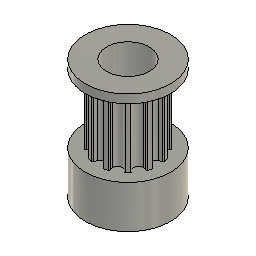
c7a76a11-5d82-49f7-98bc-9a9dc2cbd4a3 (Autodesk Fusion 360 design; units mm, degrees)
Autodesk Fusion 360 part; units mm, degrees
sketch "Sketch1" plane through (0, 0, 0) normal (0, 0, 1) x (1, 0, 0)
  arc A0 (6.2495, 2.4169) -> (6.267, 1.8336) centre (6.7302, 2.1394) ccw
  arc A1 (2.6934, 6.7634) -> (2.6052, 7.0865) centre (1.6982, 6.6655) ccw
  arc A2 (6.9322, 3.3233) -> (7.2561, 3.2381) centre (7.345, 4.2342) ccw
  arc A3 (2.4169, 1.3899) -> (1.8336, 1.3724) centre (2.1394, 0.9093) ccw
  arc A4 (3.3233, 6.9322) -> (3.8197, 6.6254) centre (3.8197, 7.1804) ccw
  arc A5 (6.2357, 6.5436) -> (6.0416, 6.5049) centre (6.1607, 6.4137) ccw
  arc A6 (4.9707, 0.3655) -> (5.0342, 0.5529) centre (4.8957, 0.4954) ccw
  arc A7 (0.5529, 5.0342) -> (0.3655, 4.9707) centre (0.4954, 4.8957) ccw
  arc A8 (3.0894, 7.3867) -> (2.6687, 7.274) centre (3.8002, 3.8925) ccw
  arc A9 (6.2495, 5.2226) -> (6.7634, 4.9461) centre (6.7302, 5.5001) ccw
  arc A10 (3.0894, 0.2527) -> (3.2381, 0.3833) centre (3.0894, 0.4027) ccw
  arc A11 (7.2561, 4.4013) -> (6.9322, 4.3161) centre (7.345, 3.4053) ccw
  arc A12 (4.4013, 0.3833) -> (4.3161, 0.7072) centre (3.4053, 0.2945) ccw
  arc A13 (7.3867, 4.5501) -> (7.274, 4.9707) centre (3.8925, 3.8392) ccw
  arc A14 (4.3161, 6.9322) -> (4.4013, 7.2561) centre (3.4053, 7.345) ccw
  arc A15 (1.8336, 1.3724) -> (1.5978, 1.1345) centre (2.416, 0.5595) ccw
  arc A16 (1.3724, 5.8059) -> (1.1345, 6.0416) centre (0.5595, 5.2234) ccw
  arc A17 (3.8197, 1.014) -> (3.3233, 0.7072) centre (3.8197, 0.459) ccw
  arc A18 (1.0958, 1.4037) -> (1.4037, 1.0958) centre (3.7664, 3.7664) ccw
  arc A19 (0.876, 2.6934) -> (0.5529, 2.6052) centre (0.974, 1.6982) ccw
  arc A20 (4.5501, 7.3867) -> (4.4013, 7.2561) centre (4.5501, 7.2367) ccw
  arc A21 (5.0342, 7.0865) -> (4.9707, 7.274) centre (4.8957, 7.1441) ccw
  arc A22 (3.2381, 7.2561) -> (3.0894, 7.3867) centre (3.0894, 7.2367) ccw
  arc A23 (1.1345, 1.5978) -> (1.3724, 1.8336) centre (0.5595, 2.416) ccw
  arc A24 (6.2357, 1.0958) -> (6.5436, 1.4037) centre (3.873, 3.7664) ccw
  arc A25 (2.6052, 0.5529) -> (2.6687, 0.3655) centre (2.7437, 0.4954) ccw
  arc A26 (1.0958, 6.2357) -> (1.1345, 6.0416) centre (1.2257, 6.1607) ccw
  arc A27 (3.3233, 0.7072) -> (3.2381, 0.3833) centre (4.2342, 0.2945) ccw
  arc A28 (1.4037, 6.5436) -> (1.0958, 6.2357) centre (3.7664, 3.873) ccw
  arc A29 (6.7634, 4.9461) -> (7.0865, 5.0342) centre (6.6655, 5.9413) ccw
  arc A30 (4.9461, 6.7634) -> (5.2226, 6.2495) centre (5.5001, 6.7302) ccw
  arc A31 (1.014, 3.8197) -> (0.7072, 4.3161) centre (0.459, 3.8197) ccw
  arc A32 (6.9322, 4.3161) -> (6.6254, 3.8197) centre (7.1804, 3.8197) ccw
  arc A33 (3.8197, 6.6254) -> (4.3161, 6.9322) centre (3.8197, 7.1804) ccw
  arc A34 (6.6254, 3.8197) -> (6.9322, 3.3233) centre (7.1804, 3.8197) ccw
  arc A35 (1.3899, 5.2226) -> (1.3724, 5.8059) centre (0.9093, 5.5001) ccw
  arc A36 (2.6934, 0.876) -> (2.4169, 1.3899) centre (2.1394, 0.9093) ccw
  arc A37 (0.5529, 5.0342) -> (0.876, 4.9461) centre (0.974, 5.9413) ccw
  arc A38 (1.3724, 1.8336) -> (1.3899, 2.4169) centre (0.9093, 2.1394) ccw
  arc A39 (0.3655, 2.6687) -> (0.5529, 2.6052) centre (0.4954, 2.7437) ccw
  arc A40 (1.5978, 6.5049) -> (1.8336, 6.267) centre (2.416, 7.0799) ccw
  arc A41 (6.5436, 1.4037) -> (6.5049, 1.5978) centre (6.4137, 1.4787) ccw
  arc A42 (0.3655, 4.9707) -> (0.2527, 4.5501) centre (3.7469, 3.8392) ccw
  arc A43 (7.274, 2.6687) -> (7.3867, 3.0894) centre (3.8925, 3.8002) ccw
  arc A44 (7.3867, 3.0894) -> (7.2561, 3.2381) centre (7.2367, 3.0894) ccw
  arc A45 (0.3833, 3.2381) -> (0.7072, 3.3233) centre (0.2945, 4.2342) ccw
  arc A46 (7.0865, 2.6052) -> (7.274, 2.6687) centre (7.1441, 2.7437) ccw
  arc A47 (0.7072, 4.3161) -> (0.3833, 4.4013) centre (0.2945, 3.4053) ccw
  arc A48 (7.2561, 4.4013) -> (7.3867, 4.5501) centre (7.2367, 4.5501) ccw
  arc A49 (5.0342, 7.0865) -> (4.9461, 6.7634) centre (5.9413, 6.6655) ccw
  arc A50 (7.0865, 2.6052) -> (6.7634, 2.6934) centre (6.6655, 1.6982) ccw
  arc A51 (4.5501, 0.2527) -> (4.9707, 0.3655) centre (3.8392, 3.7469) ccw
  arc A52 (6.7634, 2.6934) -> (6.2495, 2.4169) centre (6.7302, 2.1394) ccw
  arc A53 (5.2226, 6.2495) -> (5.8059, 6.267) centre (5.5001, 6.7302) ccw
  arc A54 (1.8336, 6.267) -> (2.4169, 6.2495) centre (2.1394, 6.7302) ccw
  arc A55 (4.9461, 0.876) -> (5.0342, 0.5529) centre (5.9413, 0.974) ccw
  circle A56 centre (3.8197, 3.8197) radius 2.5
  arc A57 (0.3833, 3.2381) -> (0.2527, 3.0894) centre (0.4027, 3.0894) ccw
  arc A58 (0.2527, 3.0894) -> (0.3655, 2.6687) centre (3.7469, 3.8002) ccw
  arc A59 (4.9707, 7.274) -> (4.5501, 7.3867) centre (3.8392, 3.8925) ccw
  arc A60 (6.0416, 1.1345) -> (5.8059, 1.3724) centre (5.2234, 0.5595) ccw
  arc A61 (4.4013, 0.3833) -> (4.5501, 0.2527) centre (4.5501, 0.4027) ccw
  arc A62 (1.1345, 1.5978) -> (1.0958, 1.4037) centre (1.2257, 1.4787) ccw
  arc A63 (3.2381, 7.2561) -> (3.3233, 6.9322) centre (4.2342, 7.345) ccw
  arc A64 (7.274, 4.9707) -> (7.0865, 5.0342) centre (7.1441, 4.8957) ccw
  arc A65 (6.267, 1.8336) -> (6.5049, 1.5978) centre (7.0799, 2.416) ccw
  arc A66 (4.3161, 0.7072) -> (3.8197, 1.014) centre (3.8197, 0.459) ccw
  arc A67 (0.2527, 4.5501) -> (0.3833, 4.4013) centre (0.4027, 4.5501) ccw
  arc A68 (1.5978, 6.5049) -> (1.4037, 6.5436) centre (1.4787, 6.4137) ccw
  arc A69 (6.267, 5.8059) -> (6.2495, 5.2226) centre (6.7302, 5.5001) ccw
  arc A70 (5.8059, 6.267) -> (6.0416, 6.5049) centre (5.2234, 7.0799) ccw
  arc A71 (0.876, 4.9461) -> (1.3899, 5.2226) centre (0.9093, 5.5001) ccw
  arc A72 (6.5436, 6.2357) -> (6.2357, 6.5436) centre (3.873, 3.873) ccw
  arc A73 (6.5049, 6.0416) -> (6.267, 5.8059) centre (7.0799, 5.2234) ccw
  arc A74 (1.3899, 2.4169) -> (0.876, 2.6934) centre (0.9093, 2.1394) ccw
  arc A75 (6.0416, 1.1345) -> (6.2357, 1.0958) centre (6.1607, 1.2257) ccw
  arc A76 (2.6687, 7.274) -> (2.6052, 7.0865) centre (2.7437, 7.1441) ccw
  arc A77 (6.5049, 6.0416) -> (6.5436, 6.2357) centre (6.4137, 6.1607) ccw
  arc A78 (0.7072, 3.3233) -> (1.014, 3.8197) centre (0.459, 3.8197) ccw
  arc A79 (2.6052, 0.5529) -> (2.6934, 0.876) centre (1.6982, 0.974) ccw
  arc A80 (5.8059, 1.3724) -> (5.2226, 1.3899) centre (5.5001, 0.9093) ccw
  arc A81 (5.2226, 1.3899) -> (4.9461, 0.876) centre (5.5001, 0.9093) ccw
  arc A82 (1.4037, 1.0958) -> (1.5978, 1.1345) centre (1.4787, 1.2257) ccw
  arc A83 (2.4169, 6.2495) -> (2.6934, 6.7634) centre (2.1394, 6.7302) ccw
  arc A84 (2.6687, 0.3655) -> (3.0894, 0.2527) centre (3.8002, 3.7469) ccw
extrude "Extrude1" add sketch "Sketch1" along normal blind 8
sketch "Sketch2" plane through (0, 0, 8) normal (0, 0, 1) x (-1, 0, 0)
  circle A0 centre (-3.8197, -3.8197) radius 2.5
  arc A1 (-2.6052, -0.5529) -> (-2.6687, -0.3655) centre (-2.7437, -0.4954) ccw
  arc A2 (-2.6687, -0.3655) -> (-3.0894, -0.2527) centre (-3.8002, -3.7469) ccw
  arc A3 (-3.0894, -0.2527) -> (-3.2381, -0.3833) centre (-3.0894, -0.4027) ccw
  arc A4 (-3.3233, -0.7072) -> (-3.2381, -0.3833) centre (-4.2342, -0.2945) ccw
  arc A5 (-4.3161, -0.7072) -> (-3.3233, -0.7072) centre (-3.8197, -0.459) ccw
  arc A6 (-4.4013, -0.3833) -> (-4.3161, -0.7072) centre (-3.4053, -0.2945) ccw
  arc A7 (-4.4013, -0.3833) -> (-4.5501, -0.2527) centre (-4.5501, -0.4027) ccw
  arc A8 (-4.5501, -0.2527) -> (-4.9707, -0.3655) centre (-3.8392, -3.7469) ccw
  arc A9 (-4.9707, -0.3655) -> (-5.0342, -0.5529) centre (-4.8957, -0.4954) ccw
  arc A10 (-4.9461, -0.876) -> (-5.0342, -0.5529) centre (-5.9413, -0.974) ccw
  arc A11 (-5.8059, -1.3724) -> (-4.9461, -0.876) centre (-5.5001, -0.9093) ccw
  arc A12 (-6.0416, -1.1345) -> (-5.8059, -1.3724) centre (-5.2234, -0.5595) ccw
  arc A13 (-6.0416, -1.1345) -> (-6.2357, -1.0958) centre (-6.1607, -1.2257) ccw
  arc A14 (-6.2357, -1.0958) -> (-6.5436, -1.4037) centre (-3.873, -3.7664) ccw
  arc A15 (-6.5436, -1.4037) -> (-6.5049, -1.5978) centre (-6.4137, -1.4787) ccw
  arc A16 (-6.267, -1.8336) -> (-6.5049, -1.5978) centre (-7.0799, -2.416) ccw
  arc A17 (-6.7634, -2.6934) -> (-6.267, -1.8336) centre (-6.7302, -2.1394) ccw
  arc A18 (-7.0865, -2.6052) -> (-6.7634, -2.6934) centre (-6.6655, -1.6982) ccw
  arc A19 (-7.0865, -2.6052) -> (-7.274, -2.6687) centre (-7.1441, -2.7437) ccw
  arc A20 (-7.274, -2.6687) -> (-7.3867, -3.0894) centre (-3.8925, -3.8002) ccw
  arc A21 (-7.3867, -3.0894) -> (-7.2561, -3.2381) centre (-7.2367, -3.0894) ccw
  arc A22 (-6.9322, -3.3233) -> (-7.2561, -3.2381) centre (-7.345, -4.2342) ccw
  arc A23 (-6.9322, -4.3161) -> (-6.9322, -3.3233) centre (-7.1804, -3.8197) ccw
  arc A24 (-7.2561, -4.4013) -> (-6.9322, -4.3161) centre (-7.345, -3.4053) ccw
  arc A25 (-7.2561, -4.4013) -> (-7.3867, -4.5501) centre (-7.2367, -4.5501) ccw
  arc A26 (-7.3867, -4.5501) -> (-7.274, -4.9707) centre (-3.8925, -3.8392) ccw
  arc A27 (-7.274, -4.9707) -> (-7.0865, -5.0342) centre (-7.1441, -4.8957) ccw
  arc A28 (-6.7634, -4.9461) -> (-7.0865, -5.0342) centre (-6.6655, -5.9413) ccw
  arc A29 (-6.267, -5.8059) -> (-6.7634, -4.9461) centre (-6.7302, -5.5001) ccw
  arc A30 (-6.5049, -6.0416) -> (-6.267, -5.8059) centre (-7.0799, -5.2234) ccw
  arc A31 (-6.5049, -6.0416) -> (-6.5436, -6.2357) centre (-6.4137, -6.1607) ccw
  arc A32 (-6.5436, -6.2357) -> (-6.2357, -6.5436) centre (-3.873, -3.873) ccw
  arc A33 (-6.2357, -6.5436) -> (-6.0416, -6.5049) centre (-6.1607, -6.4137) ccw
  arc A34 (-5.8059, -6.267) -> (-6.0416, -6.5049) centre (-5.2234, -7.0799) ccw
  arc A35 (-4.9461, -6.7634) -> (-5.8059, -6.267) centre (-5.5001, -6.7302) ccw
  arc A36 (-5.0342, -7.0865) -> (-4.9461, -6.7634) centre (-5.9413, -6.6655) ccw
  arc A37 (-5.0342, -7.0865) -> (-4.9707, -7.274) centre (-4.8957, -7.1441) ccw
  arc A38 (-4.9707, -7.274) -> (-4.5501, -7.3867) centre (-3.8392, -3.8925) ccw
  arc A39 (-4.5501, -7.3867) -> (-4.4013, -7.2561) centre (-4.5501, -7.2367) ccw
  arc A40 (-4.3161, -6.9322) -> (-4.4013, -7.2561) centre (-3.4053, -7.345) ccw
  arc A41 (-3.3233, -6.9322) -> (-4.3161, -6.9322) centre (-3.8197, -7.1804) ccw
  arc A42 (-3.2381, -7.2561) -> (-3.3233, -6.9322) centre (-4.2342, -7.345) ccw
  arc A43 (-3.2381, -7.2561) -> (-3.0894, -7.3867) centre (-3.0894, -7.2367) ccw
  arc A44 (-3.0894, -7.3867) -> (-2.6687, -7.274) centre (-3.8002, -3.8925) ccw
  arc A45 (-2.6687, -7.274) -> (-2.6052, -7.0865) centre (-2.7437, -7.1441) ccw
  arc A46 (-2.6934, -6.7634) -> (-2.6052, -7.0865) centre (-1.6982, -6.6655) ccw
  arc A47 (-1.8336, -6.267) -> (-2.6934, -6.7634) centre (-2.1394, -6.7302) ccw
  arc A48 (-1.5978, -6.5049) -> (-1.8336, -6.267) centre (-2.416, -7.0799) ccw
  arc A49 (-1.5978, -6.5049) -> (-1.4037, -6.5436) centre (-1.4787, -6.4137) ccw
  arc A50 (-1.4037, -6.5436) -> (-1.0958, -6.2357) centre (-3.7664, -3.873) ccw
  arc A51 (-1.0958, -6.2357) -> (-1.1345, -6.0416) centre (-1.2257, -6.1607) ccw
  arc A52 (-1.3724, -5.8059) -> (-1.1345, -6.0416) centre (-0.5595, -5.2234) ccw
  arc A53 (-0.876, -4.9461) -> (-1.3724, -5.8059) centre (-0.9093, -5.5001) ccw
  arc A54 (-0.5529, -5.0342) -> (-0.876, -4.9461) centre (-0.974, -5.9413) ccw
  arc A55 (-0.5529, -5.0342) -> (-0.3655, -4.9707) centre (-0.4954, -4.8957) ccw
  arc A56 (-0.3655, -4.9707) -> (-0.2527, -4.5501) centre (-3.7469, -3.8392) ccw
  arc A57 (-0.2527, -4.5501) -> (-0.3833, -4.4013) centre (-0.4027, -4.5501) ccw
  arc A58 (-0.7072, -4.3161) -> (-0.3833, -4.4013) centre (-0.2945, -3.4053) ccw
  arc A59 (-0.7072, -3.3233) -> (-0.7072, -4.3161) centre (-0.459, -3.8197) ccw
  arc A60 (-0.3833, -3.2381) -> (-0.7072, -3.3233) centre (-0.2945, -4.2342) ccw
  arc A61 (-0.3833, -3.2381) -> (-0.2527, -3.0894) centre (-0.4027, -3.0894) ccw
  arc A62 (-0.2527, -3.0894) -> (-0.3655, -2.6687) centre (-3.7469, -3.8002) ccw
  arc A63 (-0.3655, -2.6687) -> (-0.5529, -2.6052) centre (-0.4954, -2.7437) ccw
  arc A64 (-0.876, -2.6934) -> (-0.5529, -2.6052) centre (-0.974, -1.6982) ccw
  arc A65 (-1.3724, -1.8336) -> (-0.876, -2.6934) centre (-0.9093, -2.1394) ccw
  arc A66 (-1.1345, -1.5978) -> (-1.3724, -1.8336) centre (-0.5595, -2.416) ccw
  arc A67 (-1.1345, -1.5978) -> (-1.0958, -1.4037) centre (-1.2257, -1.4787) ccw
  arc A68 (-1.0958, -1.4037) -> (-1.4037, -1.0958) centre (-3.7664, -3.7664) ccw
  arc A69 (-1.4037, -1.0958) -> (-1.5978, -1.1345) centre (-1.4787, -1.2257) ccw
  arc A70 (-1.8336, -1.3724) -> (-1.5978, -1.1345) centre (-2.416, -0.5595) ccw
  arc A71 (-2.6934, -0.876) -> (-1.8336, -1.3724) centre (-2.1394, -0.9093) ccw
  arc A72 (-2.6052, -0.5529) -> (-2.6934, -0.876) centre (-1.6982, -0.974) ccw
  circle A73 centre (-3.8197, -3.8197) radius 5
  dimension "d3" = 10
  constraint concentric A0 A73
  measures "d3" diameter of A73
extrude "Extrude2" add sketch "Sketch2" along normal blind 1 contours A1 A2 A3 A4 A5 A6 A7 A8 A9 A10 A11 A12 A13 A14 A15 A16 A17 A18 A19 A20 A21 A22 A23 A24 A25 A26 A27 A28 A29 A30 A31 A32 A33 A34 A35 A36 A37 A38 A39 A40 A41 A42 A43 A44 A45 A46 A47 A48 A49 A50 A51 A52 A53 A54 A55 A56 A57 A58 A59 A60 A61 A62 A63 A64 A65 A66 A67 A68 A69 A70 A71 A72 | A73
sketch "Sketch3" plane through (0, 0, 0) normal (0, 0, -1) x (1, 0, 0)
  circle A0 centre (3.8197, -3.8197) radius 2.5
  arc A1 (2.6687, -0.3655) -> (2.6052, -0.5529) centre (2.7437, -0.4954) ccw
  arc A2 (2.6934, -0.876) -> (2.6052, -0.5529) centre (1.6982, -0.974) ccw
  arc A3 (1.8336, -1.3724) -> (2.6934, -0.876) centre (2.1394, -0.9093) ccw
  arc A4 (1.5978, -1.1345) -> (1.8336, -1.3724) centre (2.416, -0.5595) ccw
  arc A5 (1.5978, -1.1345) -> (1.4037, -1.0958) centre (1.4787, -1.2257) ccw
  arc A6 (1.4037, -1.0958) -> (1.0958, -1.4037) centre (3.7664, -3.7664) ccw
  arc A7 (1.0958, -1.4037) -> (1.1345, -1.5978) centre (1.2257, -1.4787) ccw
  arc A8 (1.3724, -1.8336) -> (1.1345, -1.5978) centre (0.5595, -2.416) ccw
  arc A9 (0.876, -2.6934) -> (1.3724, -1.8336) centre (0.9093, -2.1394) ccw
  arc A10 (0.5529, -2.6052) -> (0.876, -2.6934) centre (0.974, -1.6982) ccw
  arc A11 (0.5529, -2.6052) -> (0.3655, -2.6687) centre (0.4954, -2.7437) ccw
  arc A12 (0.3655, -2.6687) -> (0.2527, -3.0894) centre (3.7469, -3.8002) ccw
  arc A13 (0.2527, -3.0894) -> (0.3833, -3.2381) centre (0.4027, -3.0894) ccw
  arc A14 (0.7072, -3.3233) -> (0.3833, -3.2381) centre (0.2945, -4.2342) ccw
  arc A15 (0.7072, -4.3161) -> (0.7072, -3.3233) centre (0.459, -3.8197) ccw
  arc A16 (0.3833, -4.4013) -> (0.7072, -4.3161) centre (0.2945, -3.4053) ccw
  arc A17 (0.3833, -4.4013) -> (0.2527, -4.5501) centre (0.4027, -4.5501) ccw
  arc A18 (0.2527, -4.5501) -> (0.3655, -4.9707) centre (3.7469, -3.8392) ccw
  arc A19 (0.3655, -4.9707) -> (0.5529, -5.0342) centre (0.4954, -4.8957) ccw
  arc A20 (0.876, -4.9461) -> (0.5529, -5.0342) centre (0.974, -5.9413) ccw
  arc A21 (1.3724, -5.8059) -> (0.876, -4.9461) centre (0.9093, -5.5001) ccw
  arc A22 (1.1345, -6.0416) -> (1.3724, -5.8059) centre (0.5595, -5.2234) ccw
  arc A23 (1.1345, -6.0416) -> (1.0958, -6.2357) centre (1.2257, -6.1607) ccw
  arc A24 (1.0958, -6.2357) -> (1.4037, -6.5436) centre (3.7664, -3.873) ccw
  arc A25 (1.4037, -6.5436) -> (1.5978, -6.5049) centre (1.4787, -6.4137) ccw
  arc A26 (1.8336, -6.267) -> (1.5978, -6.5049) centre (2.416, -7.0799) ccw
  arc A27 (2.6934, -6.7634) -> (1.8336, -6.267) centre (2.1394, -6.7302) ccw
  arc A28 (2.6052, -7.0865) -> (2.6934, -6.7634) centre (1.6982, -6.6655) ccw
  arc A29 (2.6052, -7.0865) -> (2.6687, -7.274) centre (2.7437, -7.1441) ccw
  arc A30 (2.6687, -7.274) -> (3.0894, -7.3867) centre (3.8002, -3.8925) ccw
  arc A31 (3.0894, -7.3867) -> (3.2381, -7.2561) centre (3.0894, -7.2367) ccw
  arc A32 (3.3233, -6.9322) -> (3.2381, -7.2561) centre (4.2342, -7.345) ccw
  arc A33 (4.3161, -6.9322) -> (3.3233, -6.9322) centre (3.8197, -7.1804) ccw
  arc A34 (4.4013, -7.2561) -> (4.3161, -6.9322) centre (3.4053, -7.345) ccw
  arc A35 (4.4013, -7.2561) -> (4.5501, -7.3867) centre (4.5501, -7.2367) ccw
  arc A36 (4.5501, -7.3867) -> (4.9707, -7.274) centre (3.8392, -3.8925) ccw
  arc A37 (4.9707, -7.274) -> (5.0342, -7.0865) centre (4.8957, -7.1441) ccw
  arc A38 (4.9461, -6.7634) -> (5.0342, -7.0865) centre (5.9413, -6.6655) ccw
  arc A39 (5.8059, -6.267) -> (4.9461, -6.7634) centre (5.5001, -6.7302) ccw
  arc A40 (6.0416, -6.5049) -> (5.8059, -6.267) centre (5.2234, -7.0799) ccw
  arc A41 (6.0416, -6.5049) -> (6.2357, -6.5436) centre (6.1607, -6.4137) ccw
  arc A42 (6.2357, -6.5436) -> (6.5436, -6.2357) centre (3.873, -3.873) ccw
  arc A43 (6.5436, -6.2357) -> (6.5049, -6.0416) centre (6.4137, -6.1607) ccw
  arc A44 (6.267, -5.8059) -> (6.5049, -6.0416) centre (7.0799, -5.2234) ccw
  arc A45 (6.7634, -4.9461) -> (6.267, -5.8059) centre (6.7302, -5.5001) ccw
  arc A46 (7.0865, -5.0342) -> (6.7634, -4.9461) centre (6.6655, -5.9413) ccw
  arc A47 (7.0865, -5.0342) -> (7.274, -4.9707) centre (7.1441, -4.8957) ccw
  arc A48 (7.274, -4.9707) -> (7.3867, -4.5501) centre (3.8925, -3.8392) ccw
  arc A49 (7.3867, -4.5501) -> (7.2561, -4.4013) centre (7.2367, -4.5501) ccw
  arc A50 (6.9322, -4.3161) -> (7.2561, -4.4013) centre (7.345, -3.4053) ccw
  arc A51 (6.9322, -3.3233) -> (6.9322, -4.3161) centre (7.1804, -3.8197) ccw
  arc A52 (7.2561, -3.2381) -> (6.9322, -3.3233) centre (7.345, -4.2342) ccw
  arc A53 (7.2561, -3.2381) -> (7.3867, -3.0894) centre (7.2367, -3.0894) ccw
  arc A54 (7.3867, -3.0894) -> (7.274, -2.6687) centre (3.8925, -3.8002) ccw
  arc A55 (7.274, -2.6687) -> (7.0865, -2.6052) centre (7.1441, -2.7437) ccw
  arc A56 (6.7634, -2.6934) -> (7.0865, -2.6052) centre (6.6655, -1.6982) ccw
  arc A57 (6.267, -1.8336) -> (6.7634, -2.6934) centre (6.7302, -2.1394) ccw
  arc A58 (6.5049, -1.5978) -> (6.267, -1.8336) centre (7.0799, -2.416) ccw
  arc A59 (6.5049, -1.5978) -> (6.5436, -1.4037) centre (6.4137, -1.4787) ccw
  arc A60 (6.5436, -1.4037) -> (6.2357, -1.0958) centre (3.873, -3.7664) ccw
  arc A61 (6.2357, -1.0958) -> (6.0416, -1.1345) centre (6.1607, -1.2257) ccw
  arc A62 (5.8059, -1.3724) -> (6.0416, -1.1345) centre (5.2234, -0.5595) ccw
  arc A63 (4.9461, -0.876) -> (5.8059, -1.3724) centre (5.5001, -0.9093) ccw
  arc A64 (5.0342, -0.5529) -> (4.9461, -0.876) centre (5.9413, -0.974) ccw
  arc A65 (5.0342, -0.5529) -> (4.9707, -0.3655) centre (4.8957, -0.4954) ccw
  arc A66 (4.9707, -0.3655) -> (4.5501, -0.2527) centre (3.8392, -3.7469) ccw
  arc A67 (4.5501, -0.2527) -> (4.4013, -0.3833) centre (4.5501, -0.4027) ccw
  arc A68 (4.3161, -0.7072) -> (4.4013, -0.3833) centre (3.4053, -0.2945) ccw
  arc A69 (3.3233, -0.7072) -> (4.3161, -0.7072) centre (3.8197, -0.459) ccw
  arc A70 (3.2381, -0.3833) -> (3.3233, -0.7072) centre (4.2342, -0.2945) ccw
  arc A71 (3.2381, -0.3833) -> (3.0894, -0.2527) centre (3.0894, -0.4027) ccw
  arc A72 (3.0894, -0.2527) -> (2.6687, -0.3655) centre (3.8002, -3.7469) ccw
  circle A73 centre (3.8197, -3.8197) radius 5
  arc A74 (2.6934, -0.876) -> (2.6052, -0.5529) centre (1.6982, -0.974) ccw
  arc A75 (2.6687, -0.3655) -> (2.6052, -0.5529) centre (2.7437, -0.4954) ccw
  arc A76 (3.0894, -0.2527) -> (2.6687, -0.3655) centre (3.8002, -3.7469) ccw
  arc A77 (3.2381, -0.3833) -> (3.0894, -0.2527) centre (3.0894, -0.4027) ccw
  arc A78 (3.2381, -0.3833) -> (3.3233, -0.7072) centre (4.2342, -0.2945) ccw
  arc A79 (3.3233, -0.7072) -> (4.3161, -0.7072) centre (3.8197, -0.459) ccw
  arc A80 (4.3161, -0.7072) -> (4.4013, -0.3833) centre (3.4053, -0.2945) ccw
  arc A81 (4.5501, -0.2527) -> (4.4013, -0.3833) centre (4.5501, -0.4027) ccw
  arc A82 (4.9707, -0.3655) -> (4.5501, -0.2527) centre (3.8392, -3.7469) ccw
  arc A83 (5.0342, -0.5529) -> (4.9707, -0.3655) centre (4.8957, -0.4954) ccw
  arc A84 (5.0342, -0.5529) -> (4.9461, -0.876) centre (5.9413, -0.974) ccw
  arc A85 (4.9461, -0.876) -> (5.8059, -1.3724) centre (5.5001, -0.9093) ccw
  arc A86 (5.8059, -1.3724) -> (6.0416, -1.1345) centre (5.2234, -0.5595) ccw
  arc A87 (6.2357, -1.0958) -> (6.0416, -1.1345) centre (6.1607, -1.2257) ccw
  arc A88 (6.5436, -1.4037) -> (6.2357, -1.0958) centre (3.873, -3.7664) ccw
  arc A89 (6.5049, -1.5978) -> (6.5436, -1.4037) centre (6.4137, -1.4787) ccw
  arc A90 (6.5049, -1.5978) -> (6.267, -1.8336) centre (7.0799, -2.416) ccw
  arc A91 (6.267, -1.8336) -> (6.7634, -2.6934) centre (6.7302, -2.1394) ccw
  arc A92 (6.7634, -2.6934) -> (7.0865, -2.6052) centre (6.6655, -1.6982) ccw
  arc A93 (7.274, -2.6687) -> (7.0865, -2.6052) centre (7.1441, -2.7437) ccw
  arc A94 (7.3867, -3.0894) -> (7.274, -2.6687) centre (3.8925, -3.8002) ccw
  arc A95 (7.2561, -3.2381) -> (7.3867, -3.0894) centre (7.2367, -3.0894) ccw
  arc A96 (7.2561, -3.2381) -> (6.9322, -3.3233) centre (7.345, -4.2342) ccw
  arc A97 (6.9322, -3.3233) -> (6.9322, -4.3161) centre (7.1804, -3.8197) ccw
  arc A98 (6.9322, -4.3161) -> (7.2561, -4.4013) centre (7.345, -3.4053) ccw
  arc A99 (7.3867, -4.5501) -> (7.2561, -4.4013) centre (7.2367, -4.5501) ccw
  arc A100 (7.274, -4.9707) -> (7.3867, -4.5501) centre (3.8925, -3.8392) ccw
  arc A101 (7.0865, -5.0342) -> (7.274, -4.9707) centre (7.1441, -4.8957) ccw
  arc A102 (7.0865, -5.0342) -> (6.7634, -4.9461) centre (6.6655, -5.9413) ccw
  arc A103 (6.7634, -4.9461) -> (6.267, -5.8059) centre (6.7302, -5.5001) ccw
  arc A104 (6.267, -5.8059) -> (6.5049, -6.0416) centre (7.0799, -5.2234) ccw
  arc A105 (6.5436, -6.2357) -> (6.5049, -6.0416) centre (6.4137, -6.1607) ccw
  arc A106 (6.2357, -6.5436) -> (6.5436, -6.2357) centre (3.873, -3.873) ccw
  arc A107 (6.0416, -6.5049) -> (6.2357, -6.5436) centre (6.1607, -6.4137) ccw
  arc A108 (6.0416, -6.5049) -> (5.8059, -6.267) centre (5.2234, -7.0799) ccw
  arc A109 (5.8059, -6.267) -> (4.9461, -6.7634) centre (5.5001, -6.7302) ccw
  arc A110 (4.9461, -6.7634) -> (5.0342, -7.0865) centre (5.9413, -6.6655) ccw
  arc A111 (4.9707, -7.274) -> (5.0342, -7.0865) centre (4.8957, -7.1441) ccw
  arc A112 (4.5501, -7.3867) -> (4.9707, -7.274) centre (3.8392, -3.8925) ccw
  arc A113 (4.4013, -7.2561) -> (4.5501, -7.3867) centre (4.5501, -7.2367) ccw
  arc A114 (4.4013, -7.2561) -> (4.3161, -6.9322) centre (3.4053, -7.345) ccw
  arc A115 (4.3161, -6.9322) -> (3.3233, -6.9322) centre (3.8197, -7.1804) ccw
  arc A116 (3.3233, -6.9322) -> (3.2381, -7.2561) centre (4.2342, -7.345) ccw
  arc A117 (3.0894, -7.3867) -> (3.2381, -7.2561) centre (3.0894, -7.2367) ccw
  arc A118 (2.6687, -7.274) -> (3.0894, -7.3867) centre (3.8002, -3.8925) ccw
  arc A119 (2.6052, -7.0865) -> (2.6687, -7.274) centre (2.7437, -7.1441) ccw
  arc A120 (2.6052, -7.0865) -> (2.6934, -6.7634) centre (1.6982, -6.6655) ccw
  arc A121 (2.6934, -6.7634) -> (1.8336, -6.267) centre (2.1394, -6.7302) ccw
  arc A122 (1.8336, -6.267) -> (1.5978, -6.5049) centre (2.416, -7.0799) ccw
  arc A123 (1.4037, -6.5436) -> (1.5978, -6.5049) centre (1.4787, -6.4137) ccw
  arc A124 (1.0958, -6.2357) -> (1.4037, -6.5436) centre (3.7664, -3.873) ccw
  arc A125 (1.1345, -6.0416) -> (1.0958, -6.2357) centre (1.2257, -6.1607) ccw
  arc A126 (1.1345, -6.0416) -> (1.3724, -5.8059) centre (0.5595, -5.2234) ccw
  arc A127 (1.3724, -5.8059) -> (0.876, -4.9461) centre (0.9093, -5.5001) ccw
  arc A128 (0.876, -4.9461) -> (0.5529, -5.0342) centre (0.974, -5.9413) ccw
  arc A129 (0.3655, -4.9707) -> (0.5529, -5.0342) centre (0.4954, -4.8957) ccw
  arc A130 (0.2527, -4.5501) -> (0.3655, -4.9707) centre (3.7469, -3.8392) ccw
  arc A131 (0.3833, -4.4013) -> (0.2527, -4.5501) centre (0.4027, -4.5501) ccw
  arc A132 (0.3833, -4.4013) -> (0.7072, -4.3161) centre (0.2945, -3.4053) ccw
  arc A133 (0.7072, -4.3161) -> (0.7072, -3.3233) centre (0.459, -3.8197) ccw
  arc A134 (0.7072, -3.3233) -> (0.3833, -3.2381) centre (0.2945, -4.2342) ccw
  arc A135 (0.2527, -3.0894) -> (0.3833, -3.2381) centre (0.4027, -3.0894) ccw
  arc A136 (0.3655, -2.6687) -> (0.2527, -3.0894) centre (3.7469, -3.8002) ccw
  arc A137 (0.5529, -2.6052) -> (0.3655, -2.6687) centre (0.4954, -2.7437) ccw
  arc A138 (0.5529, -2.6052) -> (0.876, -2.6934) centre (0.974, -1.6982) ccw
  arc A139 (0.876, -2.6934) -> (1.3724, -1.8336) centre (0.9093, -2.1394) ccw
  arc A140 (1.3724, -1.8336) -> (1.1345, -1.5978) centre (0.5595, -2.416) ccw
  arc A141 (1.0958, -1.4037) -> (1.1345, -1.5978) centre (1.2257, -1.4787) ccw
  arc A142 (1.4037, -1.0958) -> (1.0958, -1.4037) centre (3.7664, -3.7664) ccw
  arc A143 (1.5978, -1.1345) -> (1.4037, -1.0958) centre (1.4787, -1.2257) ccw
  arc A144 (1.5978, -1.1345) -> (1.8336, -1.3724) centre (2.416, -0.5595) ccw
  arc A145 (1.8336, -1.3724) -> (2.6934, -0.876) centre (2.1394, -0.9093) ccw
extrude "Extrude3" add sketch "Sketch3" along normal blind 5 contours A1 A2 A3 A4 A5 A6 A7 A8 A9 A10 A11 A12 A13 A14 A15 A16 A17 A18 A19 A20 A21 A22 A23 A24 A25 A26 A27 A28 A29 A30 A31 A32 A33 A34 A35 A36 A37 A38 A39 A40 A41 A42 A43 A44 A45 A46 A47 A48 A49 A50 A51 A52 A53 A54 A55 A56 A57 A58 A59 A60 A61 A62 A63 A64 A65 A66 A67 A68 A69 A70 A71 A72 A74 A75 A76 A77 A78 A79 A80 A81 A82 A83 A84 A85 A86 A87 A88 A89 A90 A91 A92 A93 A94 A95 A96 A97 A98 A99 A100 A101 A102 A103 A104 A105 A106 A107 A108 A109 A110 A111 A112 A113 A114 A115 A116 A117 A118 A119 A120 A121 A122 A123 A124 A125 A126 A127 A128 A129 A130 A131 A132 A133 A134 A135 A136 A137 A138 A139 A140 A141 A142 A143 A144 A145 | A73
